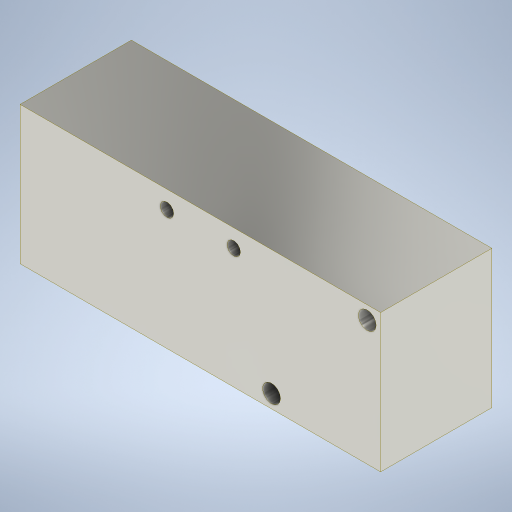
# Autodesk Inventor part: Bluepill
Saved by Autodesk Inventor 2023 (Build 270158000, 158)
## iProperties
Created: 2023-04-14
Part Number: Bluepill
Material: Silver
Document SubType Name: Modeling
Designer: Timothée
Density: 10.49 g/cm^3
Appearance: Silver
Author: Timothée
Autodesk Inventor part; units mm, degrees
ref_plane "YZ Plane" through (0, 0, 0) normal (1, 0, 0) x (0, 1, 0)
ref_plane "XZ Plane" through (0, 0, 0) normal (0, 1, 0) x (-1, 0, 0)
ref_plane "XY Plane" through (0, 0, 0) normal (0, 0, 1) x (1, 0, 0)
sketch "Sketch1" plane through (0, 0, 0) normal (0, 0, 1) x (1, 0, 0)
  line L0 (-40.5, -15.5) -> (40.5, -15.5)
  line L1 (40.5, -15.5) -> (40.5, 15.5)
  line L2 (40.5, 15.5) -> (-40.5, 15.5)
  line L3 (-40.5, 15.5) -> (-40.5, -15.5)
  line L4 (-40.5, -15.5) -> (40.5, 15.5) construction
  line L5 (40.5, -15.5) -> (-40.5, 15.5) construction
  line L6 (37.5, 15.5) -> (37.5, -15.5)
  circle A0 centre (37.5, 12.5) radius 2
  line L7 (16, -15.5) -> (16, 15.5)
  circle A1 centre (16, -12.5) radius 2
  line L8 (7.5, -15.5) -> (7.5, 15.5)
  circle A2 centre (7.5, 11.5) radius 1.5
  line L9 (-7.5, -15.5) -> (-7.5, 15.5)
  circle A3 centre (-7.5, 11.5) radius 1.5
  point P0 (0, 0)
  dimension "d0" = 3
  dimension "d1" = 81
  dimension "d2" = 31
  dimension "d3" = 4
  dimension "d4" = 3
  dimension "d5" = 24.5
  dimension "d6" = 4
  dimension "d7" = 3
  dimension "d8" = 30
  dimension "d9" = 3
  dimension "d11" = 4
  dimension "d12" = 15
  dimension "d13" = 3
  constraints: 20 end point, 12 point on line, 5 perpendicular, 4 centre point, 2 midpoint, 2 parallel, 1 horizontal
  measures "d0" distance between parallel lines of L1 L6
  measures "d1" distance of L1.end L2.end
  measures "d2" distance of L0.end L1.end
  measures "d3" diameter of A0
  measures "d4" distance from line of L2 A0.centre
  measures "d5" distance between parallel lines of L1 L7
  measures "d6" diameter of A1
  measures "d7" distance of L7.start A1.centre
  measures "d8" distance from line of A0.centre L8
  measures "d9" diameter of A2
  measures "d11" distance from line of L2 A2.centre
  measures "d12" distance between parallel lines of L8 L9
  measures "d13" diameter of A3
extrude "Extrusion1" add sketch "Sketch1" along normal blind 25 contours L3 L2 L9 A3 L0 | L9 A3 L2 L8 A2 L0 | L8 A2 L2 L7 A1 L0 | L7 A1 L2 L6 A0 L0 | L6 A0 L2 L1 L0
body "Solid1"
